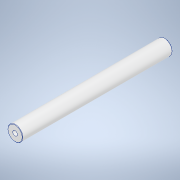
# Autodesk Inventor part: 軸_8-80
Saved by Autodesk Inventor 2021 (Build 250183000, 183)
## iProperties
Created: 2022-02-03
Part Number: 軸_8-80
Material: アルミニウム 6061
Document SubType Name: Modeling
Designer: hirohumi
Density: 2.7 g/cm^3
Appearance: アルミニウム - フラット
Author: hirohumi
Autodesk Inventor part; units mm, degrees
ref_plane "YZ Plane" through (0, 0, 0) normal (1, 0, 0) x (0, 1, 0)
ref_plane "XZ Plane" through (0, 0, 0) normal (0, 1, 0) x (-1, 0, 0)
ref_plane "XY Plane" through (0, 0, 0) normal (0, 0, 1) x (1, 0, 0)
sketch "スケッチ1" plane through (0, 0, 0) normal (0, 0, 1) x (1, 0, 0)
  circle A0 centre (0, 0) radius 4
  circle A1 centre (0, 0) radius 1.25
  dimension "d0" = 8
  dimension "d1" = 2.5
  constraints: 2 centre point, 2 coincident
  measures "d0" diameter of A0
  measures "d1" diameter of A1
extrude "押し出し1" add sketch "スケッチ1" along normal blind 80
chamfer "面取り1" distance 0.2 angle 45 2 edges at (-4, 0, 0) (-4, 0, 80)
